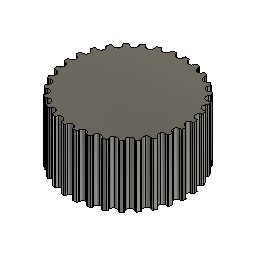
gear_31z (Autodesk Fusion 360 design; units mm, degrees)
Autodesk Fusion 360 part; units mm, degrees
sketch "Sketch1" plane through (0, 0, 0) normal (0, 0, 1) x (1, 0, 0) in component "gt2 pulley"
  circle A0 centre (0, 0) radius 9.8676 construction
  circle A1 centre (0, 0) radius 8.8636 construction
  line L0 (0, 0) -> (0, 9.8676) construction
  line L1 (0, 0) -> (0.9983, 9.817) construction
  line L2 (0, 0) -> (1.41, 9.7664) construction
  circle A2 centre (0, 0) radius 9.6136 construction
  arc A3 (0.3748, 9.468) -> (0.428, 9.1898) centre (1.3737, 9.515) ccw
  circle A4 centre (0, 0) radius 9.4636 construction
  arc A5 (0.2285, 9.6109) -> (0, 9.6136) centre (0, 0) ccw
  arc A6 (0.3748, 9.468) -> (0.2285, 9.6109) centre (0.225, 9.4609) ccw
  arc A7 (0.428, 9.1898) -> (0.8967, 8.8181) centre (0.9529, 9.3703) ccw
  arc A8 (0, 9.6136) -> (-0.2285, 9.6109) centre (0, 0) ccw
  arc A9 (-0.2285, 9.6109) -> (-0.3748, 9.468) centre (-0.225, 9.4609) ccw
  arc A10 (-0.428, 9.1898) -> (-0.3748, 9.468) centre (-1.3737, 9.515) ccw
  arc A11 (-0.8971, 8.8181) -> (-0.428, 9.1898) centre (-0.9529, 9.3703) ccw
  arc A12 (0.8967, 8.8181) -> (-0.8967, 8.8181) centre (0, 0) ccw
  point P0 (1.3737, 9.515)
  point P1 (0, 9.6136)
  dimension "d18" = 19.7352
  dimension "d19" = 5.806
  dimension "d22" = 1.004
  dimension "d24" = 0.75
  dimension "d26" = 1
  dimension "d27" = 0.15
  dimension "d28" = 0.15
  dimension "d47" = 0.555
  dimension "d52" = 3.812
  constraint coincident A0.centre A1.centre
  constraint coincident A0 L0.end
  constraint vertical L0
  constraint coincident A0 L1.end
  constraint coincident A0 L2.end
  constraint concentric A1 A2
  constraint coincident A1 A7.end
  constraint coincident L1 A7.end
  constraint coincident A2 P0
  constraint coincident L2 P0
  constraint coincident P0 A3.centre
  constraint coincident A2 P1
  constraint coincident L0 P1
  constraint concentric A2 A4
  constraint coincident P1 A5.end
  constraint coincident A4 A6.centre
  constraint coincident A3.start A6.start
  constraint tangent A3 A6
  constraint tangent A3 A7
  constraint symmetric L0 A7.end A12.end
  constraint symmetric L0 A3.start A9.end
  constraint symmetric L0 A3.end A10.start
  constraint symmetric L0 A3 A10
  constraint symmetric L0 A5.start A8.end
  constraint symmetric L0 P1 A5.end
  constraint symmetric L0 A5 A8
  constraint symmetric L0 A6 A9
  constraint symmetric L0 A7 A11
  constraint coincident A1 A11.start
  constraint tangent A1 A7
  constraint coincident L1 A7.centre
  measures "d18" diameter of A0
  measures "d19" angle of L0 L1
  measures "d22" distance of A0 A1
  measures "d24" distance of A1 A2
  measures "d26" radius of A3
  measures "d27" distance of A2 A4
  measures "d28" radius of A6
  measures "d47" radius of A7
extrude "Extrude1" add sketch "Sketch1" along normal blind 10 makes body 1
pattern_circular "C-Pattern1" count 31 over 360 about axis through (0, 0, 1.75) along (0, 0, 1) of bodies 1 makes body 2 at (-1.0951, 8.7957, 3.3333) makes body 3 at (-3.5871, 8.1053, 6.6667) makes body 4 at (-5.1453, 7.2173, 6.6667) makes body 5 at (-5.9235, 6.5936, 3.3333) makes body 6 at (-7.1295, 5.2662, 3.3333) makes body 7 at (-8.5286, 2.414, 6.6667) makes body 8 at (-8.776, 1.2432, 6.6667) makes body 9 at (-8.8466, -0.5488, 6.6667) makes body 10 at (-8.7289, -1.5392, 3.3333) makes body 11 at (-8.2404, -3.2648, 3.3333) makes body 12 at (-6.9474, -5.5042, 6.6667) makes body 13 at (-6.2851, -6.2499, 3.3333) makes body 14 at (-4.8984, -7.3871, 3.3333) makes body 15 at (-3.3111, -8.2219, 3.3333) makes body 16 at (-1.5882, -8.7202, 3.3333) makes body 17 at (1.5886, -8.7201, 6.6667) makes body 18 at (3.3115, -8.2218, 6.6667) makes body 19 at (3.678, -8.0645, 3.3333) makes body 20 at (6.2854, -6.2496, 6.6667) makes body 21 at (6.5602, -5.9605, 3.3333) makes body 22 at (8.0013, -3.8134, 6.6667) makes body 23 at (8.729, -1.5388, 6.6667) makes body 24 at (8.8567, -0.349, 6.6667) makes body 25 at (8.8399, 0.6482, 3.3333) makes body 26 at (8.5284, 2.4144, 3.3333) makes body 27 at (7.8678, 4.0817, 3.3333) makes body 28 at (6.8851, 5.582, 3.3333) makes body 29 at (4.4746, 7.6512, 6.6667) makes body 30 at (4.1259, 7.8448, 3.3333) makes body 31 at (2.4623, 8.5147, 3.3333)
sketch "Sketch2" plane through (0, 0, 10) normal (0, 0, 1) x (-1, 0, 0)
  arc A0 (-5.7164, -7.5569) -> (-5.6779, -7.7578) centre (-5.5894, -7.6367) ccw
  arc A1 (-5.6779, -7.7578) -> (-5.3029, -8.0188) centre (0, 0) ccw
  arc A2 (-5.3029, -8.0188) -> (-5.1011, -7.9851) centre (-5.2201, -7.8937) ccw
  arc A3 (-4.8986, -7.7872) -> (-5.1011, -7.9851) centre (-4.3081, -8.5943) ccw
  arc A4 (-4.3015, -7.7499) -> (-4.8986, -7.7872) centre (-4.5709, -8.2351) ccw
  arc A5 (-5.7735, -6.7253) -> (-4.3015, -7.7499) centre (0, 0) ccw
  arc A6 (-5.6012, -7.2982) -> (-5.7735, -6.7253) centre (-6.135, -7.1464) ccw
  arc A7 (-5.7164, -7.5569) -> (-5.6012, -7.2982) centre (-6.5631, -7.0248) ccw
  circle A8 centre (0, 0) radius 8.8636
  constraint concentric A1 A8
extrude "Extrude2" add sketch "Sketch2" against normal blind 10 contours A5 A8 bodies 1 2 3 4 5 6 7 8 9 10 11 12 13 14 15 16 17 18 19 20 21 22 23 24 25 26 27 28 29 30 31
extrude "Extrude4" [suppressed] in component "gt2 pulley"
pattern_circular "C-Pattern7" [suppressed] in component "gt2 pulley"
extrude "Extrude3" [suppressed] in component "gt2 pulley"
pattern_circular "C-Pattern6" [suppressed] in component "gt2 pulley"
extrude "Extrude2'" [suppressed] in component "gt2 pulley"
pattern_circular "C-Pattern5" [suppressed] in component "gt2 pulley"
extrude "Extrude1'" [suppressed] in component "gt2 pulley"
pattern_circular "C-Pattern4" [suppressed] in component "gt2 pulley"
pattern_circular "C-Pattern3" [suppressed] in component "gt2 pulley"
pattern_circular "C-Pattern2" [suppressed] in component "gt2 pulley"
pattern_circular "C-Pattern1'" [suppressed] in component "gt2 pulley"
copy_body "Body->Comp1" [suppressed] in component "Component"
copy_body "Body->Comp2" [suppressed] in component "Component'"
copy_body "Body->Comp3" [suppressed] in component "Component''"
copy_body "Body->Comp4" [suppressed] in component "Component'''"
copy_body "Body->Comp5" [suppressed] in component "Component''''"
copy_body "Body->Comp6" [suppressed] in component "Component'''''"
copy_body "Body->Comp7" [suppressed] in component "Component''''''"
copy_body "Body->Comp8" [suppressed] in component "Component'''''''"
copy_body "Body->Comp9" [suppressed] in component "Component''''''''"
copy_body "Body->Comp10" [suppressed] in component "Component'''''''''"
copy_body "Body->Comp11" [suppressed] in component "Component''''''''''"
copy_body "Body->Comp12" [suppressed] in component "Component'''''''''''"
copy_body "Body->Comp13" [suppressed] in component "Component''''''''''''"
copy_body "Body->Comp14" [suppressed] in component "Component'''''''''''''"
copy_body "Body->Comp15" [suppressed] in component "Component''''''''''''''"
copy_body "Body->Comp16" [suppressed] in component "Component'''''''''''''''"
copy_body "Body->Comp17" [suppressed] in component "Component''''''''''''''''"
copy_body "Body->Comp18" [suppressed] in component "Component'''''''''''''''''"
copy_body "Body->Comp19" [suppressed] in component "Component''''''''''''''''''"
copy_body "Body->Comp20" [suppressed] in component "Component'''''''''''''''''''"
component "gt2 pulley" placed x (1, 0, 0) y (0, 1, 0) z (0, 0, 1) at (0, 0, 0)
equation "NumTeeth = 31" comment "min 20"
equation "ToothPitch = 2 mm"
equation "PullyDia = NumTeeth * ToothPitch / PI"
equation "ToothAng = ( ( 360 / NumTeeth ) * 1 deg )"
equation "TransOffsetAngle = ToothAng * 0.2"
equation "Sholulder_Radius = 0.15 mm"
equation "Root_Radius = 0.555 mm"
equation "TransRadius = 1 mm"
equation "ToolHeight = 0.75 mm"
equation "PLD = 0.254 mm"
equation "d18 = PullyDia"
equation "d19 = ToothAng / 2"
equation "d22 = PLD + ToolHeight"
equation "d24 = ToolHeight"
equation "d26 = TransRadius"
equation "d27 = Sholulder_Radius"
equation "d31 = NumTeeth"
equation "d33 = NumTeeth"
equation "d35 = NumTeeth"
equation "d37 = NumTeeth"
equation "d41 = NumTeeth"
equation "d45 = NumTeeth"
equation "d47 = Root_Radius"
equation "d50 = NumTeeth"
